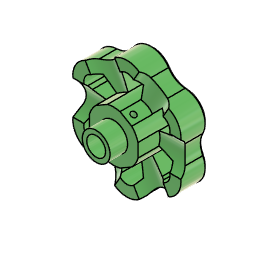
VerticalDrillFrame v27 (Autodesk Fusion 360 archive; units mm, degrees)
design "Knob_58"
Autodesk Fusion 360 part; units mm, degrees
sketch "Sketch1" plane through (0, 0, 0) normal (0, 1, 0) x (1, 0, 0) in component "58mm"
  circle A0 centre (0, 0) radius 27 construction
  circle A1 centre (0, 0) radius 11.5
  circle A2 centre (0, 0) radius 6.35
  circle A3 centre (0, 0) radius 4.3
  line L0 (0, 0) -> (0, -27)
  line L1 (0, 0) -> (-13.5, -23.3827)
  line L2 (0, 0) -> (13.5, -23.3827)
  line L3 (6.9881, -26.08) -> (0, 0)
  line L4 (-6.9881, -26.08) -> (0, 0)
  arc A4 (11.2604, -19.5035) -> (8.0052, -22.6154) centre (16.0104, -27.7308) ccw
  arc A5 (-8.0052, -22.6154) -> (-11.2604, -19.5035) centre (-16.0104, -27.7308) ccw
  arc A6 (-8.0052, -22.6154) -> (8.0052, -22.6154) centre (0, -17.5) ccw
  arc A7 (8.7604, -15.1734) -> (3.7919, -19.9231) centre (16.0104, -27.7308) ccw
  arc A8 (-3.7919, -19.9231) -> (3.7919, -19.9231) centre (0, -17.5) ccw
  arc A9 (-3.7919, -19.9231) -> (-8.7604, -15.1734) centre (-16.0104, -27.7308) ccw
  dimension "d10_1" = 54
  dimension "d11_1" = 23
  dimension "d12_1" = 12.7
  dimension "d13_1" = 8.6
  dimension "d16_1" = 30
  dimension "d17_1" = 30
  dimension "d18_1" = 15
  dimension "d20_1" = 9.5
  dimension "d21_1" = 15
  dimension "d22_1" = 9.5
  dimension "d23_1" = -5
  constraint concentric A0 A1
  constraint concentric A1 A2
  constraint concentric A2 A3
  constraint coincident A0.centre A1.centre
  constraint vertical L0
  constraint coincident L2 A4.start
  constraint coincident A0 L3.start
  constraint coincident L2 A4.centre
  constraint symmetric L0 A4.end A5.start
  constraint symmetric L0 A4.start A5.end
  constraint symmetric L0 A4 A5
  constraint coincident A0 L4.start
  constraint tangent A0 A6
  constraint tangent A4 A6
  constraint coincident A0 L0.end
  constraint coincident A0 L2.end
  constraint coincident A0 L1.end
  measures "d10_1" diameter of A0
  measures "d11_1" diameter of A1
  measures "d12_1" diameter of A2
  measures "d13_1" diameter of A3
  measures "d16_1" angle of L0 L1
  measures "d17_1" angle of L0 L2
  measures "d18_1" angle of L0 L3
  measures "d20_1" radius of A4
  measures "d21_1" angle of L0 L4
  measures "d22_1" radius of A6
extrude "Extrude1" add sketch "Sketch1" against normal blind 12 contours A1 L1 L4 A9 | A1 L2 L3 A7 | L1 L4 A5 A6 A9 | L2 L3 A4 A6 A7 | L0 L4 A6 A8 A9 | L0 L3 A6 A7 A8 makes body 1 in component "58mm"
pattern_circular "C-Pattern1" count 6 over 360 about axis through (0, 1.75, 0) along (0, 1, 0) of "Extrude1" makes body 2 at (9.8699, 0, 12.4801) makes body 3 at (15.743, 0, -2.3076) makes body 4 at (5.8731, 0, -14.7876) makes body 5 at (-9.8699, 0, -12.4801) makes body 6 at (-15.743, 0, 2.3076) in component "58mm"
extrude "Extrude2" add sketch "Sketch1" against normal blind 18 contours A1 A2 L1 L2 | A1 A2 L1 L4 | A1 A2 L2 L3 | A1 A2 L0 L4 | A1 A2 L0 L3 bodies 1 2 3 4 5 6 in component "58mm"
extrude "Extrude3" add sketch "Sketch1" against normal blind 26 contours A2 A3 L1 L4 | A2 A3 L1 L2 | A2 A3 L2 L3 | A2 A3 L0 L4 | A2 A3 L0 L3 bodies 1 in component "58mm"
sketch "Sketch2" plane through (0, 0, 0) normal (1, 0, 0) x (0, 1, 0) in component "58mm"
  circle A0 centre (-17.5, 0) radius 9.5
  circle A1 centre (-14.5, 0) radius 3.3305
  circle A2 centre (-14.5, 0) radius 2.159 construction
  circle A3 centre (-14.5, 0) radius 1.25
  dimension "d32_1" = 19
  dimension "d33_1" = 6.6611
  dimension "d34_1" = 4.318
  dimension "d35_1" = 2.5
  dimension "d36_1" = 14.5
  dimension "d37_1" = 17.5
  constraint horizontal origin A0.centre
  constraint horizontal origin A1.centre
  constraint concentric A1 A2
  constraint concentric A2 A3
  measures "d32_1" diameter of A0
  measures "d33_1" diameter of A1
  measures "d34_1" diameter of A2
  measures "d35_1" diameter of A3
  measures "d36_1" distance of origin A1.centre
  measures "d37_1" distance of origin A0.centre
extrude "Extrude4" cut sketch "Sketch2" along normal blind -11.0771 and the other way blind 41.0781 contours A0 | A1 | A3 bodies 1 in component "58mm"
pattern_circular "C-Pattern2" count 6 over 360 about axis through (0, 1.75, 0) along (0, 1, 0) of "Extrude4" in component "58mm"
extrude "Extrude6" cut sketch "Sketch2" against normal blind 11.3255 contours A3 bodies 1 in component "58mm"
pattern_circular "C-Pattern3" count 3 over 360 about axis through (0, 1.75, 0) along (0, 1, 0) of "Extrude6" in component "58mm"
fillet "Fillet2" [suppressed] in component "58mm"
chamfer "Chamfer1" distance 1 angle 45 12 edges at (-11.2604, 0, 19.5035) (-23.3827, 0, 13.5) (-22.5207, 0, 0) (-23.3827, 0, -13.5) (-11.2604, 0, -19.5035) (0, 0, -27) (11.2604, 0, -19.5035) (23.3827, 0, -13.5) (22.5207, 0, 0) (23.3827, 0, 13.5) (11.2604, 0, 19.5035) (0, 0, 27) on bodies 1 in component "58mm"
sketch "Sketch1 (2)" plane through (0, 0, 0) normal (0, 1, 0) x (1, 0, 0) in component "Lock"
  circle A0 centre (0, 0) radius 4
  circle A1 centre (0, 0) radius 10
  line L0 (0, 0) -> (10, 0)
  line L1 (0, 0) -> (0, 10)
  line L2 (0, 1.65) -> (10, 1.65)
  line L3 (1.65, 0) -> (1.65, 10)
  line L4 (10, 1.65) -> (10, 0)
  line L5 (0, 10) -> (1.65, 10)
  dimension "d1" = 8
  dimension "d2" = 6
  dimension "d5" = -1.65
  dimension "d6" = 10
  dimension "d7" = 1.65
  dimension "d8" = 10
  constraint coincident A0.centre A1.centre
  constraint coincident A1 L0.end
  constraint horizontal L0
  constraint coincident A1 L1.end
  constraint perpendicular L0 L1
  constraint coincident L1 L2.start
  constraint coincident L0 L3.start
  measures "d1" diameter of A0
  measures "d6" distance of L2.start L2.end
  measures "d8" distance of L3.start L3.end
extrude "Extrude1'" add sketch "Sketch1 (2)" along normal mid plane 6 separate body contours A0 A1 L0 L1 | A0 A1 L0 L2 | A0 A1 L2 L3 | A0 A1 L1 L3 makes body 7 in component "Lock"
revolve "Revolve1" cut sketch "Sketch1 (2)" angle 360 about axis through (0, 0, 0) along (1, 0, 0) contours A0 A1 L0 L2 | A1 L2 L4 bodies 7 in component "Lock"
revolve "Revolve2" cut sketch "Sketch1 (2)" angle 360 about axis through (0, 0, 0) along (0, 0, -1) contours A0 A1 L1 L3 | A1 L3 L5 bodies 7 in component "Lock"
component "58mm" placed x (1, 0, 0) y (0, 1, 0) z (0, 0, 1) at (0, 0, 0)
component "Lock" placed x (1, 0, 0) y (0, 1, 0) z (0, 0, 1) at (0, 0, 0)
equation "d17_1 = d16_1"
equation "d21_1 = d18_1"

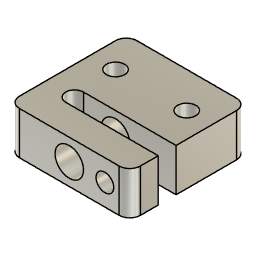
design "TR8x2_Nut"
Autodesk Fusion 360 part; units mm, degrees
sketch "Sketch1" plane through (0, 0, 0) normal (0, 0, 1) x (1, 0, 0) in component "TR8x2_Nut"
  line L0 (17, 16.5) -> (-17, 16.5)
  line L1 (-17, 16.5) -> (-17, -16.5)
  line L2 (-17, -16.5) -> (17, -16.5)
  line L3 (17, -16.5) -> (17, 16.5)
  line L4 (17, 16.5) -> (-17, -16.5) construction
  line L5 (-17, 16.5) -> (17, -16.5) construction
  line L6 (-9, -8.5) -> (17, -8.5)
  line L7 (-9, -3.5) -> (17, -3.5)
  line L8 (-17, 6.5) -> (17, 6.5) construction
  line L9 (-9, -8.5) -> (-9, -3.5) construction
  arc A0 (-9, -3.5) -> (-9, -8.5) centre (-9, -6) ccw
  circle A1 centre (-10, 6.5) radius 2.55
  line L10 (0, 0) -> (0, 16.5) construction
  circle A2 centre (10, 6.5) radius 2.55
  dimension "d1" = 34
  dimension "d2" = 33
  dimension "d7" = 26
  dimension "d8" = 5.1
  dimension "d9" = 7
  dimension "d10" = 10
  dimension "d11" = 20
  dimension "d12" = 5
  constraint horizontal L0
  constraint perpendicular L0 L1
  constraint parallel L1 L3
  constraint coincident L4 L10.start
  constraint coincident L5 L10.start
  constraint coincident L10.start origin
  constraint parallel L2 L6
  constraint parallel L2 L7
  constraint parallel L2 L8
  constraint coincident L3 L6.end
  constraint coincident L3 L7.end
  constraint coincident L3 L8.end
  constraint coincident L1 L8.start
  constraint perpendicular L7 L9
  constraint midpoint L9 A0.centre
  constraint coincident L8 A1.centre
  constraint midpoint L0 L10.end
  constraint symmetric A1 L10 A2
  measures "d1" distance of L1.end L2.end
  measures "d2" distance of L0.end L1.end
  measures "d7" distance of L3 L9
  measures "d8" diameter of A1
  measures "d9" distance of L1 A1.centre
  measures "d10" distance of L0 L8
  measures "d11" distance of L0 L7
  measures "d12" distance of L6 L7
extrude "Extrude1" add sketch "Sketch1" along normal mid plane 12 contours L0 L1 L2 L3 L6 L7 A0 in component "TR8x2_Nut"
sketch "Sketch2" plane through (0, 0, 0) normal (0, 1, 0) x (1, 0, 0) in component "TR8x2_Nut"
  circle A0 centre (0, 0) radius 4
  circle A1 centre (10, 0) radius 2.5
  dimension "d15" = 8
  dimension "d16" = 5
  dimension "d17" = 10
  constraint coincident A0.centre origin
  constraint horizontal A0.centre A1.centre
  measures "d15" diameter of A0
  measures "d16" diameter of A1
  measures "d17" distance of A0.centre A1.centre
extrude "Extrude2" cut sketch "Sketch2" against normal blind 12.9576 from surface at -8.5 contours A1 in component "TR8x2_Nut"
extrude "Extrude3" cut sketch "Sketch2" along normal mid plane 84.5817 contours A0 in component "TR8x2_Nut"
fillet "Fillet1" radius 3 4 edges at (-17, -16.5, 0) (17, -16.5, 0) (17, 16.5, 0) (-17, 16.5, 0) in component "TR8x2_Nut"
component "TR8x2_Nut" placed x (1, 0, 0) y (0, 1, 0) z (0, 0, 1) at (0, 0, 0)
